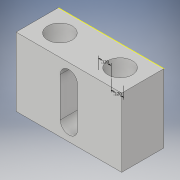
# Autodesk Inventor part: Hew Sensor Mount 2017
Saved by Autodesk Inventor 2017 (Build 210142000, 142)
## iProperties
Created: 2016-10-05
Part Number: Hew Sensor Mount 2017
Material: Generic
Document SubType Name: Sheet Metal
Designer: situh
Density: 1 g/cm^3
Sheet Metal Rule: Default
Appearance: Default
Author: situh
Autodesk Inventor part; units mm, degrees
ref_plane "YZ Plane" through (0, 0, 0) normal (1, 0, 0) x (0, 1, 0)
ref_plane "XZ Plane" through (0, 0, 0) normal (0, 1, 0) x (-1, 0, 0)
ref_plane "XY Plane" through (0, 0, 0) normal (0, 0, 1) x (1, 0, 0)
sketch "Sketch1" plane through (0, 0, 0) normal (0, 0, 1) x (1, 0, 0)
  line L0 (-6.2599, 9.5475) -> (19.1401, 9.5475)
  line L1 (19.1401, 9.5475) -> (19.1401, -6.9625)
  line L2 (19.1401, -6.9625) -> (-6.2599, -6.9625)
  line L3 (-6.2599, -6.9625) -> (-6.2599, 9.5475)
  point P0 (0, 0)
  dimension "d0" = 25.4
  dimension "d1" = 16.51
  measures "d0" distance of L0.start L0.end
  measures "d1" distance of L2.end L0.start
extrude "Plate1" add sketch "Sketch1" along normal blind 10.16
sketch "Sketch4" plane through (-6.2599, -6.9625, 0) normal (0, -1, 0) x (1, 0, 0)
  circle A0 centre (5.461, 5.08) radius 2.4765
  circle A1 centre (19.939, 5.08) radius 2.4765
  line L0 (25.4, 0) -> (25.4, 10.16) projected
  line L1 (0, 0) -> (0, 10.16) projected
  line L2 (25.4, 10.16) -> (0, 10.16) projected
  circle A2 centre (5.461, 5.08) radius 2.4765
  circle A3 centre (19.939, 5.08) radius 2.4765
  dimension "d30" = 4.953
  dimension "d37" = 5.461
  dimension "d38" = 5.461
  constraints: 4 centre point, 2 coincident, 2 concentric
  measures "d30" diameter of A0
  measures "d37" distance from line of L1 A0.centre
  measures "d38" distance from line of L0 A1.centre
extrude "Extrusion1" cut sketch "Sketch4" against normal blind 14
sketch "Sketch5" plane through (-6.2599, 9.5475, 0) normal (0, 1, 0) x (1, 0, 0)
  circle A0 centre (5.461, -5.08) radius 2.4765 projected
  circle A1 centre (5.461, -5.08) radius 2.9464
  circle A2 centre (19.939, -5.08) radius 2.4765 projected
  circle A3 centre (19.939, -5.08) radius 2.9464
  line L0 (25.4, 0) -> (25.4, -10.16) projected
  line L1 (0, 0) -> (0, -10.16) projected
  point P0 (6.2599, 0)
  constraints: 2 centre point, 2 coincident
extrude "Extrusion2" cut sketch "Sketch5" against normal blind 10
sketch "Sketch6" plane through (0, 0, 0) normal (0, 0, -1) x (-1, 0, 0)
  line L0 (-19.1401, 9.5475) -> (-19.1401, -6.9625) projected
  line L1 (6.2599, 9.5475) -> (-19.1401, 9.5475)
  line L2 (6.2599, -6.9625) -> (6.2599, 9.5475) projected
  line L3 (6.2599, 1.2925) -> (-19.1401, 1.2925) construction
  line L4 (-6.4401, 6.0296) -> (-6.4401, -3.4446) construction
  line L5 (-19.1401, -6.9625) -> (6.2599, -6.9625) projected
  line L6 (-8.5229, 6.0296) -> (-8.5229, -3.4446)
  line L7 (-4.3573, -3.4446) -> (-4.3573, 6.0296)
  arc A0 (-4.3573, 6.0296) -> (-8.5229, 6.0296) centre (-6.4401, 6.0296) ccw
  arc A1 (-8.5229, -3.4446) -> (-4.3573, -3.4446) centre (-6.4401, -3.4446) ccw
  point P0 (-6.4401, 1.2925)
  dimension "d26" = 13.6398
  dimension "d27" = 2.0828
  constraints: 12 end point, 4 midpoint, 4 point on circle, 4 tangent, 2 centre point, 1 parallel, 1 perpendicular
  measures "d27" radius of A1
extrude "Extrusion3" cut sketch "Sketch6" against normal through all contours A0 L7 A1 L6
sketch "Sketch7" plane through (-6.2599, 9.5475, 0) normal (0, 1, 0) x (1, 0, 0)
  circle A0 centre (5.461, -5.08) radius 2.9464 projected
  circle A1 centre (5.461, -5.08) radius 2.4765
  circle A2 centre (19.939, -5.08) radius 2.4765 projected
  circle A3 centre (19.939, -5.08) radius 2.4765
  point P0 (6.2599, 0)
  constraints: 2 centre point, 2 coincident
extrude "Extrusion4" cut sketch "Sketch7" against normal up to next contours A1 | A2
sketch "Sketch8" plane through (0, 0, 0) normal (0, 0, -1) x (-1, 0, 0)
  arc A0 (-8.5229, -3.4446) -> (-4.3573, -3.4446) centre (-6.4401, -3.4446) ccw projected
  line L0 (-8.5229, -3.4446) -> (-8.5229, 6.0296) projected
  line L1 (-6.4401, 1.2925) -> (-3.3921, 1.2925) construction
  line L2 (-6.4401, 1.2925) -> (-9.4881, 1.2925) construction
  line L3 (-3.3921, 1.2925) -> (-3.3921, 9.5475) construction
  line L4 (6.2599, 9.5475) -> (-19.1401, 9.5475) projected
  point P0 (0, 0)
  dimension "d41" = 3.048
  dimension "d42" = 3.048
  constraints: 6 end point, 1 horizontal, 1 perpendicular, 1 point on line, 1 vertical
  measures "d41" distance of L1.start L1.end
  measures "d42" distance of L1.start L2.end
equation "\"BendRadius\" = Thickness"
equation "\"BendReliefWidth\" = Thickness"
equation "\"BendReliefDepth\" = 0.5 * Thickness"
equation "\"CornerReliefSize\" = 4 * Thickness"
equation "\"MinimumRemnant\" = 2 * Thickness"
equation "\"TransitionRadius\" = BendRadius"
equation "\"JacobiRadiusSize\" = Thickness"
equation "\"GapSize\" = Thickness"
equation "\"d2\" = BendRadius"
equation "\"Thickness\" = 10.16"
body "Solid1"
